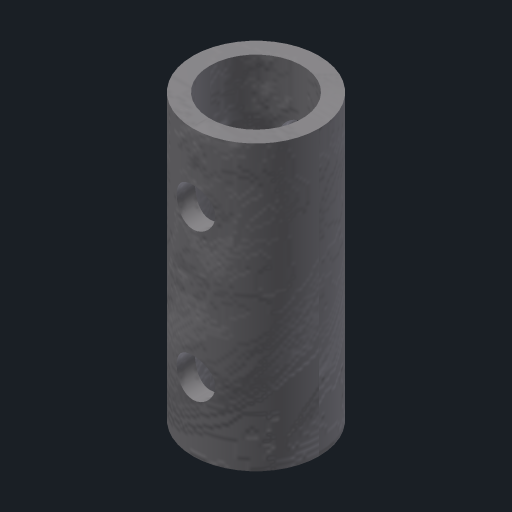
# Autodesk Inventor part: ACOMPLE_PLASTICO
Saved by Autodesk Inventor 2024.3 (Build 283343000, 343)
## iProperties
Created: 2024-07-01
Part Number: ACOMPLE_PLASTICO
Material: Steel, Mild, Welded
Document SubType Name: Modeling
Designer: Niler
Density: 7.85 g/cm^3
Appearance: Weld - Steel Mild
Author: Niler
Autodesk Inventor part; units mm, degrees
ref_plane "YZ Plane" through (0, 0, 0) normal (1, 0, 0) x (0, 1, 0)
ref_plane "XZ Plane" through (0, 0, 0) normal (0, 1, 0) x (-1, 0, 0)
ref_plane "XY Plane" through (0, 0, 0) normal (0, 0, 1) x (1, 0, 0)
sketch "Sketch1" plane through (0, 0, 0) normal (0, 1, 0) x (-1, 0, 0)
  circle A0 centre (0, 0) radius 5.55
  circle A1 centre (0, 0) radius 4.05
  dimension "d0" = 11.1
  dimension "d1" = 8.1
  constraints: 2 centre point, 2 coincident
  measures "d0" diameter of A0
  measures "d1" diameter of A1
extrude "Extrusion1" add sketch "Sketch1" along normal blind 25
sketch "Sketch2" plane through (0, 0, 0) normal (0, 0, 1) x (1, 0, 0)
  line L0 (5.55, 25) -> (-5.55, 25) projected
  line L1 (5.55, 0) -> (-5.55, 0) projected
  circle A0 centre (0, 6) radius 1.7
  line L2 (5.55, 0) -> (-5.55, 0) projected
  line L3 (-4.05, 25) -> (-4.05, 0) projected
  circle A1 centre (0, 19) radius 1.7
  point P0 (0, 0)
  point P1 (0, 25)
  dimension "d4" = 3.4
  dimension "d5" = 6
  dimension "d6" = 3.4
  dimension "d7" = 6
  constraints: 2 centre point, 2 vertical alignment, 1 midpoint
  measures "d4" diameter of A0
  measures "d5" distance of A0.centre point (0, 0)
  measures "d6" diameter of A1
  measures "d7" distance from line of L0 A1.centre
extrude "Extrusion2" cut sketch "Sketch2" along normal mid plane 25
body "Solid1"
